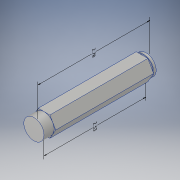
# Autodesk Inventor part: ARM_010_2.75inHexShaft
Saved by Autodesk Inventor 2018 (Build 220112000, 112)
## iProperties
Created: 2019-01-22
Part Number: ARM_010_2.75inHexShaft
Material: Aluminum 6061
Document SubType Name: Modeling
Designer: carls
Mass: 131.24 g
Surface Area: 156.563 cm^2
Volume: 48.6075 cm^3
Density: 2.7 g/cm^3
Appearance: Aluminum - Flat
Author: carls
Autodesk Inventor part; units mm, degrees
ref_plane "YZ Plane" through (0, 0, 0) normal (1, 0, 0) x (0, 1, 0)
ref_plane "XZ Plane" through (0, 0, 0) normal (0, 1, 0) x (-1, 0, 0)
ref_plane "XY Plane" through (0, 0, 0) normal (0, 0, 1) x (1, 0, 0)
sketch "Sketch1" plane through (0, 0, 0) normal (0, 0, 1) x (1, 0, 0)
  line L0 (7.3323, 0) -> (3.6662, -6.35)
  line L1 (3.6662, -6.35) -> (-3.6662, -6.35)
  line L2 (-3.6662, -6.35) -> (-7.3323, 0)
  line L3 (-7.3323, 0) -> (-3.6662, 6.35)
  line L4 (-3.6662, 6.35) -> (3.6662, 6.35)
  line L5 (3.6662, 6.35) -> (7.3323, 0)
  point P0 (0, 0)
  point P1 (0, 0)
  dimension "d0" = 12.7
  constraints: 12 end point, 1 coincident, 13 other
  measures "d0" distance between parallel lines of L1 L4
extrude "Extrusion1" add sketch "Sketch1" along normal mid plane 343.535
sketch "Sketch2" plane through (0, 0, 171.7675) normal (0, 0, 1) x (1, 0, 0)
  circle A0 centre (0, 0) radius 5.9436
  dimension "d3" = 11.8872
  constraints: 1 centre point, 1 coincident
  measures "d3" diameter of A0
extrude "Extrusion2" add sketch "Sketch2" along normal blind 0.9906
sketch "Sketch3" plane through (0, 0, 172.7581) normal (0, 0, 1) x (1, 0, 0)
  circle A0 centre (0, 0) radius 5.9436 projected
  line L0 (3.6662, -6.35) -> (7.3323, 0) projected
  line L1 (7.3323, 0) -> (3.6662, 6.35) projected
  line L2 (3.6662, 6.35) -> (-3.6662, 6.35) projected
  line L3 (-3.6662, 6.35) -> (-7.3323, 0) projected
  line L4 (-7.3323, 0) -> (-3.6662, -6.35) projected
  line L5 (-3.6662, -6.35) -> (3.6662, -6.35) projected
  circle A1 centre (0, 0) radius 6.35
  constraints: 1 centre point, 1 coincident
extrude "Extrusion3" add sketch "Sketch3" along normal blind 1.5875 contours A0 | A1
mirror "Mirror1" about plane through (0, 0, 0) normal (0, 0, 1) of "Extrusion2", "Extrusion3"
sketch "Sketch4" plane through (-3.6662, -6.35, -171.7675) normal (-0.866, -0.5, 0) x (0, 0, 1)
  line L0 (61.571, -23.211) -> (381.4095, -23.211)
  line L1 (381.4095, -23.211) -> (381.4095, 34.5749)
  line L2 (381.4095, 34.5749) -> (61.571, 34.5749)
  line L3 (61.571, 34.5749) -> (61.571, -23.211)
  point P0 (171.7675, 3.6662)
  constraints: 8 end point, 2 parallel, 1 horizontal, 1 perpendicular
extrude "Extrusion4" cut sketch "Sketch4" against normal blind 25.4
sketch "Sketch5" plane through (-3.6662, -6.35, -110.1965) normal (0, 0, 1) x (1, 0, 0)
  circle A0 centre (3.6662, 6.35) radius 6.35
  dimension "d10" = 12.7
  constraints: 1 centre point, 1 coincident
  measures "d10" diameter of A0
extrude "Extrusion5" add sketch "Sketch5" along normal blind 6.35
body "Solid1"
